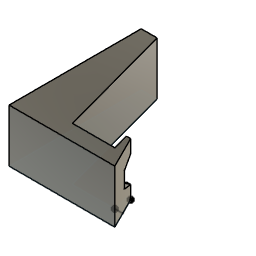
Spring-Holder v1 (Autodesk Fusion 360 design; units mm, degrees)
part number: Konfiguration 1
Autodesk Fusion 360 part; units mm, degrees
sketch "Skizze1" plane through (0, 0, 0) normal (0, 0, 1) x (1, 0, 0)
  line L0 (0, 0) -> (0, 25)
  line L1 (0, 0) -> (20, 0)
  line L2 (0, 25) -> (3, 25)
  line L3 (17, 3) -> (9, 3)
  line L4 (3, 25) -> (9, 3)
  line L5 (3, 25) -> (3, 3) construction
  line L6 (3, 3) -> (9, 3) construction
  line L7 (17, 6) -> (20, 0)
  line L8 (17, 6) -> (16.1818, 6)
  line L9 (17, 3) -> (16.1818, 6)
  line L10 (17, 3) -> (22, 3) construction
  dimension "d1" = 3
  dimension "d4" = 74.745
  dimension "d5" = 105.255
  constraint coincident L0.start L1.start
  constraint vertical L0
  constraint perpendicular L0 L1
  constraint perpendicular L0 L2
  constraint perpendicular L2 L5
  constraint perpendicular L5 L6
  constraint horizontal L10
  measures "d1" distance of L0.end L2.end
  measures "d4" angle of L4 L6
  measures "d5" angle of L9 L10
extrude "Extrusion1" add sketch "Skizze1" along normal blind 10
sketch "Skizze3" plane through (0, 0, 0) normal (0, 0, -1) x (1, 0, 0)
  line L0 (20, 0) -> (0, 0)
  line L1 (0, 0) -> (0, -25)
  line L2 (0, -25) -> (3, -25)
  line L3 (3, -25) -> (9, -3)
  line L4 (9, -3) -> (17, -3)
  line L5 (17, -3) -> (16.1818, -6)
  line L6 (16.1818, -6) -> (17, -6)
  line L7 (17, -6) -> (20, 0)
  line L8 (17, -3) -> (18.5, -3)
  line L9 (18.5, -3) -> (17, -6) construction
  constraint coincident L4.end L5.start
  constraint midpoint L7 L8.end
  constraint coincident L6.end L7.start
sketch "Skizze4" plane through (16, 8, 0) normal (0.894427, 0.447214, 0) x (-0.447214, 0.894427, 0)
  line L0 (-8.9443, 0) -> (-2.2361, 0)
  line L1 (-2.2361, 0) -> (-2.2361, 10)
  line L2 (-2.2361, 10) -> (-8.9443, 10)
  line L3 (-8.9443, 10) -> (-8.9443, 0)
  line L4 (-8.9443, 10) -> (-8.9443, 0) construction
  line L5 (-8.9443, 5) -> (-2.2361, 5) construction
  line L6 (-8.9443, 2.5) -> (-2.2361, 2.5) construction
  line L7 (-8.9443, 7.5) -> (-2.2361, 7.5) construction
  line L8 (-2.2361, 7.5) -> (-8.9443, 5)
  line L9 (-2.2361, 2.5) -> (-8.9443, 5)
  line L10 (-2.2361, 0) -> (-5.5902, 0) construction
  line L11 (-5.5902, 0) -> (-5.5902, 10) construction
  line L12 (-5.5902, 3.75) -> (-5.5902, 6.25)
  dimension "d10" = 2.5
  dimension "d11" = 2.5
  dimension "d13" = 3.3541
  dimension "d14" = 6.7082
  constraint coincident L2.end L3.start
  constraint coincident L0.start L3.end
  constraint midpoint L3 L5.start
  constraint midpoint L1 L5.end
  constraint coincident L3 L6.start
  constraint coincident L1 L6.end
  constraint perpendicular L1 L6
  constraint coincident L3 L7.start
  constraint coincident L1 L7.end
  constraint perpendicular L3 L7
  constraint coincident L0.end L1.start
  constraint perpendicular L1 L10
  constraint perpendicular L7 L11
  constraint midpoint L9 L12.start
  constraint midpoint L8 L12.end
  measures "d10" distance of L5 L6
  measures "d11" distance of L5 L7
  measures "d13" distance of L0.end L10.end
  measures "d14" distance of L1.end L2.end
extrude "Extrusion2" cut sketch "Skizze4" against normal blind 1.5 contours L1 L8 L9 L12
extrude "Extrusion3" cut 1 faces at (16.52, 5.76, 5.8333) along direction (-0.447214, 0.894427, 0) blind 0.4
extrude "Extrusion4" add 1 faces at (16.9348, 2.7764, 4.5833) along direction (0.894427, 0.447214, 0) blind 1.5
equation "d5 = 180 deg - 74.7448809423 deg"
